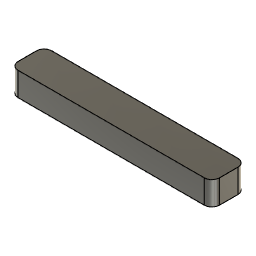
MiserSpoolPin (Autodesk Fusion 360 design; units mm, degrees)
Autodesk Fusion 360 part; units mm, degrees
sketch "Sketch1" plane through (0, 0, 0) normal (0, 0, 1) x (1, 0, 0)
  line L0 (0, 0) -> (40, 0)
  line L1 (40, 0) -> (40, 6)
  line L2 (40, 6) -> (0, 6)
  line L3 (0, 6) -> (0, 0)
  dimension "d1" = 40
  dimension "d2" = 6
  constraint horizontal L0
  constraint vertical L1
  constraint horizontal L2
  constraint vertical L3
  constraint coincident L0.start L3.end
  measures "d1" distance of L0.start L0.end
  measures "d2" distance of L0.start L2.end
extrude "Extrude1" add sketch "Sketch1" along normal blind 4
extrude "Extrude2" add 1 faces at (26.6667, 6, 1.3333) along direction (0, 1, 0) blind 0.7
extrude "Extrude3" add 1 faces at (13.3333, 4.4667, 4) along direction (0, 0, 1) blind 0.7
fillet "Fillet1" radius 1.5 4 edges at (0, 6.7, 2.35) (0, 0, 2.35) (40, 0, 2.35) (40, 6.7, 2.35)
